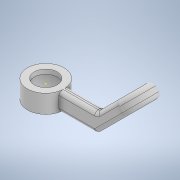
# Autodesk Inventor part: Skrzynia-dol-ramie
Saved by Autodesk Inventor 2022 (Build 260153000, 153)
## iProperties
Created: 2022-03-27
Part Number: Skrzynia-dol-ramie
Material: Ogólny
Document SubType Name: Modeling
Designer: jolow
Density: 1 g/cm^3
Appearance: Domyślna
Author: jolow
Autodesk Inventor part; units mm, degrees
ref_plane "YZ Plane" through (0, 0, 0) normal (1, 0, 0) x (0, 1, 0)
ref_plane "XZ Plane" through (0, 0, 0) normal (0, 1, 0) x (-1, 0, 0)
ref_plane "XY Plane" through (0, 0, 0) normal (0, 0, 1) x (1, 0, 0)
sketch "Szkic1" plane through (0, 0, 0) normal (0, 1, 0) x (-1, 0, 0)
  circle A0 centre (0, 0) radius 20
  dimension "d0" = 40
  constraints: 1 centre point, 1 coincident
  measures "d0" diameter of A0
extrude "Wyciągnięcie proste1" add sketch "Szkic1" along normal mid plane 20
sketch "Szkic2" plane through (0, 0, 0) normal (0, 0, 1) x (1, 0, 0)
  line L0 (-20, -10) -> (20, -10) projected
  line L1 (0, -10) -> (60, -10)
  line L2 (60, -10) -> (60, 10)
  line L3 (60, 10) -> (0, 10)
  line L4 (0, 10) -> (0, -10)
  line L5 (60, 10) -> (97, 47)
  line L6 (97, 47) -> (107, 37)
  line L7 (107, 37) -> (60, -10)
  line L8 (0, 10) -> (0, 144)
  line L9 (0, 144) -> (97, 47)
  point P0 (0, 0)
  dimension "d3" = 20
  dimension "d4" = 45
  dimension "d5" = 134
  dimension "d6" = 60
  constraints: 18 end point, 3 parallel, 3 perpendicular, 1 horizontal, 1 midpoint, 1 vertical
  measures "d3" distance of L1.end L2.end
  measures "d4" angle of L9 L8
  measures "d5" distance of L3.end L8.end
  measures "d6" distance of L2.end L3.end
extrude "Wyciągnięcie proste2" add sketch "Szkic2" along normal mid plane 10 contours L4 L3 L2 L1 L0 | L2 L5 L6 L7
sketch "Szkic3" plane through (60, 10, -5) normal (-0.7071068, 0.7071068, 0) x (-0.7071068, -0.7071068, 0)
  line L0 (-52.3259, 0) -> (-52.3259, 10) projected
  circle A0 centre (-52.3259, 5) radius 11
  circle A1 centre (-52.3259, 5) radius 16
  point P0 (49.4975, 5)
  dimension "d9" = 22
  dimension "d10" = 5
  constraints: 2 centre point, 1 coincident, 1 midpoint
  measures "d9" diameter of A0
  measures "d10" radial gap between concentric circles of A1 A0
extrude "Wyciągnięcie proste3" add sketch "Szkic3" against normal up to surface (14.1421 mm away)
sketch "Szkic4" plane through (60, 10, -5) normal (-0.7071068, 0.7071068, 0) x (-0.7071068, -0.7071068, 0)
  line L0 (-52.3259, 0) -> (-52.3259, 10) projected
  circle A0 centre (-52.3259, 5) radius 11
  point P0 (49.4975, 5)
  constraints: 1 centre point, 1 midpoint
extrude "Wyciągnięcie proste4" cut sketch "Szkic4" against normal through all
sketch "Szkic5" plane through (0, -10, 0) normal (0, -1, 0) x (1, 0, 0)
  circle A0 centre (0, 0) radius 15
  dimension "d15" = 30
  constraints: 1 centre point, 1 coincident
  measures "d15" diameter of A0
extrude "Wyciągnięcie proste5" cut sketch "Szkic5" against normal through all
fillet "Zaokrąglenie2" radius 4 11 edges at (39.6825, 10, 5) (39.6825, 10, -5) (60, 10, 0) (73.1265, 23.1265, -5) (73.1265, 23.1265, 5) (39.6825, -10, 5) (39.6825, -10, -5) (78.1265, 8.1265, 5) (60, -10, 0) (78.1265, 8.1265, -5) (118.3137, 48.3137, 0)
sketch "Szkic6" plane through (0, 10, 0) normal (0, 1, 0) x (1, 0, 0)
  circle A0 centre (0, 0) radius 15
  constraints: 1 centre point, 1 coincident
extrude "Wyciągnięcie proste6" add sketch "Szkic6" against normal blind 5
sketch "Szkic7" plane through (0, 10, 0) normal (0, 1, 0) x (1, 0, 0)
  circle A0 centre (0, 0) radius 12.5
  dimension "d22" = 25
  constraints: 1 centre point, 1 coincident
  measures "d22" diameter of A0
extrude "Wyciągnięcie proste7" cut sketch "Szkic7" against normal blind 5
fillet "Zaokrąglenie3" radius 5 1 edges at (108.3137, 58.3137, 0)
sketch "Szkic8" plane through (0, 5, 0) normal (0, -1, 0) x (1, 0, 0)
  point P0 (0, 0)
